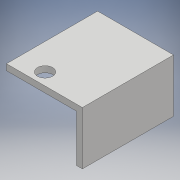
# Autodesk Inventor part: ブレーキ固定アングル
Saved by Autodesk Inventor 2018 (Build 220112000, 112)
## iProperties
Created: 2017-10-14
Part Number: ブレーキ固定アングル
Material: 一般
Document SubType Name: Modeling
Designer: mura5
Density: 1 g/cm^3
Appearance: 既定
Author: mura5
Autodesk Inventor part; units mm, degrees
ref_plane "YZ Plane" through (0, 0, 0) normal (1, 0, 0) x (0, 1, 0)
ref_plane "XZ Plane" through (0, 0, 0) normal (0, 1, 0) x (-1, 0, 0)
ref_plane "XY Plane" through (0, 0, 0) normal (0, 0, 1) x (1, 0, 0)
sketch "スケッチ1" plane through (0, 0, 0) normal (0, 1, 0) x (-1, 0, 0)
  line L0 (0, 0) -> (0, -35)
  line L1 (0, -35) -> (4, -35)
  line L2 (4, -35) -> (4, -4)
  line L3 (4, -4) -> (50, -4)
  line L4 (50, -4) -> (50, 0)
  line L5 (50, 0) -> (0, 0)
  dimension "d0" = 35
  dimension "d1" = 4
  dimension "d2" = 90
  dimension "d3" = 31
  dimension "d4" = 46
  constraints: 12 end point, 5 perpendicular, 1 vertical
  measures "d0" distance of L0.start L0.end
  measures "d1" distance of L0.end L1.end
  measures "d2" angle of L1 L0
  measures "d3" distance of L1.end L2.end
  measures "d4" distance of L2.end L3.end
extrude "押し出し1" add sketch "スケッチ1" along normal blind 60
sketch "スケッチ2" plane through (-50, 0, 0) normal (0, 0, 1) x (1, 0, 0)
  line L0 (50, 0) -> (50, 60) projected
  line L1 (0, 0) -> (50, 0) projected
  point P0 (17.3731, 8.0322)
  dimension "d7" = 32.6269
  dimension "d8" = 8.0322
  measures "d7" distance from line of L0 point (17.373, 8.032)
  measures "d8" distance from line of point (17.373, 8.032) L1
hole "穴1" at (-32.6269, 8.0322, 0) direction (0, 0, -1) diameter 10 end through all
